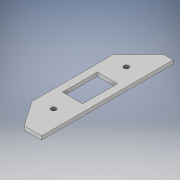
# Autodesk Inventor part: orginal_headplate_ben
Saved by Autodesk Inventor 2017 (Build 210142000, 142)
## iProperties
Created: 2017-02-24
Part Number: orginal_headplate_ben
Material: Generic
Document SubType Name: Modeling
Designer: richp
Density: 1 g/cm^3
Appearance: Default
mounting_hole_distance: 1.248 in
Author: richp
Autodesk Inventor part; units mm, degrees
ref_plane "YZ Plane" through (0, 0, 0) normal (1, 0, 0) x (0, 1, 0)
ref_plane "XZ Plane" through (0, 0, 0) normal (0, 1, 0) x (-1, 0, 0)
ref_plane "XY Plane" through (0, 0, 0) normal (0, 0, 1) x (1, 0, 0)
sketch "Sketch1" plane through (0, 0, 0) normal (0, 1, 0) x (-1, 0, 0)
  line L0 (-7.5692, 28.702) -> (7.5692, 28.702) construction
  line L1 (7.5692, 28.702) -> (7.5692, -28.702) construction
  line L2 (7.5692, -28.702) -> (-7.5692, -28.702) construction
  line L3 (-7.5692, -28.702) -> (-7.5692, 28.702) construction
  line L4 (-7.5692, 28.702) -> (7.5692, -28.702) construction
  line L5 (7.5692, 28.702) -> (-7.5692, -28.702) construction
  line L6 (-4.3815, -7.5692) -> (4.3815, -7.5692)
  line L7 (4.3815, -7.5692) -> (4.3815, 7.5692)
  line L8 (4.3815, 7.5692) -> (-4.3815, 7.5692)
  line L9 (-4.3815, 7.5692) -> (-4.3815, -7.5692)
  line L10 (-4.3815, -7.5692) -> (4.3815, 7.5692) construction
  line L11 (4.3815, -7.5692) -> (-4.3815, 7.5692) construction
  line L12 (-7.5692, -28.702) -> (-3.3782, -28.702)
  line L13 (7.5692, -17.78) -> (-3.3782, -28.702)
  line L14 (-7.5692, -28.702) -> (-7.5692, 0)
  line L15 (21.6792, 0) -> (-18.0822, 0) construction
  line L16 (-7.5692, 28.702) -> (-7.5692, 0)
  line L17 (7.5692, 0) -> (7.5692, -17.78)
  line L18 (7.5692, 0) -> (7.5692, 17.78)
  line L19 (-7.5692, 28.702) -> (0, 28.702)
  line L20 (7.5692, 17.78) -> (0, 28.702)
  point P0 (0, 0)
  point P1 (0, -15.8496)
  point P2 (0, 15.8496)
  point P3 (0, 0)
  dimension "d0" = 57.404
  dimension "d1" = 15.1384
  dimension "d2" = 8.763
  dimension "d3" = 15.1384
  dimension "d4" = 10.9474
  dimension "d5" = 10.922
  dimension "d7" = 7.5692
  dimension "d20" = 10.922
  dimension "d21" = 7.5692
  dimension "mounting_hole_distance" = 31.6992
  constraints: 42 end point, 8 midpoint, 4 parallel, 4 point on line, 3 horizontal, 2 perpendicular, 1 collinear, 1 symmetric about line
  measures "d0" distance of L0.end L1.end
  measures "d1" distance of L0.start L0.end
  measures "d2" distance of L7.end L8.end
  measures "d3" distance of L6.end L7.end
  measures "d4" horizontal distance of L13.start L12.end
  measures "d5" vertical distance of L13.start L12.end
  measures "d7" distance from line of L1 point (0, -15.85)
  measures "d20" vertical distance of L18.end L19.end
  measures "d21" horizontal distance of L18.end L19.end
  measures "mounting_hole_distance" distance of point (0, 15.85) point (0, -15.85)
extrude "Extrusion2" add sketch "Sketch1" against normal blind 1.5748
hole "Hole1" at (0, 0, -15.8496) at (0, 0, 15.8496) direction (0, -1, 0) diameter 2.159 depth 8.8646 tip angle 118
equation "\"d20\" = d5"
equation "\"d21\" = d7"
body "Solid2"
